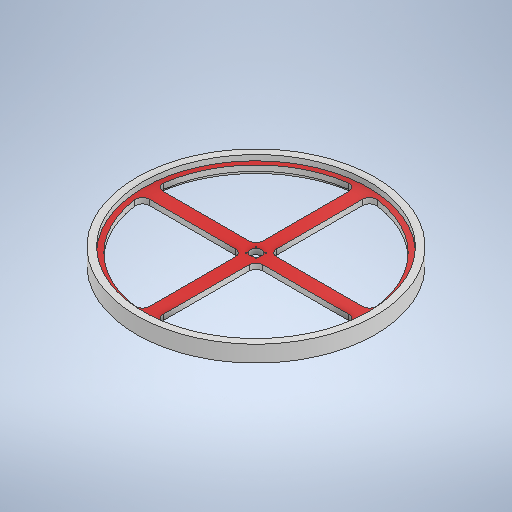
# Autodesk Inventor part: 05
Saved by Autodesk Inventor 2025.1 (Build 291241000, 241)
## iProperties
Created: 2024-09-17
Part Number: 05
Material: Generisch
Document SubType Name: Modeling
Designer: ffogue
Density: 1 g/cm^3
Appearance: Vorgabe
Author: ffogue
Autodesk Inventor part; units mm, degrees
ref_plane "YZ Plane" through (0, 0, 0) normal (1, 0, 0) x (0, 1, 0)
ref_plane "XZ Plane" through (0, 0, 0) normal (0, 1, 0) x (-1, 0, 0)
sketch "Sketch1" plane through (0, 0, 0) normal (0, 0, 1) x (1, 0, 0)
  circle A0 centre (0, 0) radius 175
  dimension "d0" = 350
  constraints: 1 centre point, 1 coincident
  measures "d0" diameter of A0
extrude "Extrusion1" add sketch "Sketch1" along normal mid plane 24
sketch "Sketch2" plane through (0, 0, 12) normal (0, 0, 1) x (1, 0, 0)
  circle A0 centre (0, 0) radius 165
  dimension "d3" = 330
  constraints: 1 centre point, 1 coincident
  measures "d3" diameter of A0
extrude "Extrusion2" cut sketch "Sketch2" against normal blind 8
ref_plane "Work Plane1" through (0, 0, 0) normal (0, 0, 1) x (1, 0, 0)
mirror "Mirror1" about plane through (0, 0, 0) normal (0, 0, 1) of "Extrusion2"
sketch "Sketch3" plane through (0, 0, 4) normal (0, 0, 1) x (1, 0, 0)
  circle A0 centre (0, 0) radius 8
  line L0 (-10, -10) -> (-10, -157.1822)
  line L1 (10, -10) -> (10, -157.1822)
  line L2 (0, 0) -> (0, -162.7163) construction
  arc A1 (-157.1822, -10) -> (-10, -157.1822) centre (0, 0) ccw
  line L3 (-10, -10) -> (-157.1822, -10)
  arc A2 (10, -157.1822) -> (157.1822, -10) centre (0, 0) ccw
  line L4 (10, -10) -> (157.1822, -10)
  dimension "d7" = 16
  dimension "d8" = 20
  dimension "d9" = 157.5
  dimension "d10" = 10
  constraints: 10 end point, 4 point on circle, 3 centre point, 3 coincident, 3 vertical, 2 horizontal, 2 horizontal alignment, 1 other
  measures "d7" diameter of A0
  measures "d8" distance between parallel lines of L1 L0
  measures "d9" radius of A1
  measures "d10" distance from line of L3 point (0, 0)
extrude "Extrusion3" cut sketch "Sketch3" against normal blind 8 contours L0 A1 L3 | L4 A2 L1
pattern_circular "Circular Pattern1" count 2 over 360 about axis through (0, 0, 12) along (0, 0, -1) of "Extrusion3"
fillet "Fillet1" radius 10 12 edges at (-10, 157.1822, 0) (-157.1822, 10, 0) (-10, 10, 0) (-10, -10, 0) (-157.1822, -10, 0) (-10, -157.1822, 0) (10, -157.1822, 0) (10, -10, 0) (157.1822, -10, 0) (157.1822, 10, 0) (10, 10, 0) (10, 157.1822, 0)
extrude "Extrusion4" cut sketch "Sketch3" against normal up to surface (8 mm away) contours A0
sketch "Sketch4" plane through (0, 0, 4) normal (0, 0, 1) x (1, 0, 0)
  circle A0 centre (0, 0) radius 8 projected
  circle A1 centre (0, 0) radius 10 construction
  line L0 (0, 0) -> (-7.0711, 7.0711) construction
  line L1 (0, 0) -> (0, 20.2635) construction
  dimension "d21" = 20
  dimension "d22" = 45
  constraints: 4 end point, 2 coincident, 1 vertical, 3 other
  measures "d22" angle of L1 L0
hole "Hole1" at (-7.0711, 7.0711, 4) direction (0, 0, -1) diameter 2 depth 8
pattern_circular "Circular Pattern2" count 4 over 360 about axis through (0, 0, 4) along (0, 0, -1) of "Hole1"
body "Solid1"
